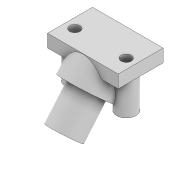
# Autodesk Inventor part: Landing_leg_clamp_large
Saved by Autodesk Inventor 2022 (Build 260153000, 153)
## iProperties
Created: 2022-05-01
Part Number: Landing_leg_clamp_large
Material: Generic
Document SubType Name: Modeling
Designer: dell
Density: 1 g/cm^3
Appearance: Default
Mass: 2.35409 g
Surface Area: 17.5445 cm^2
Volume: 2.35409 cm^3
Author: dell
Autodesk Inventor part; units mm, degrees
ref_plane "YZ Plane" through (0, 0, 0) normal (1, 0, 0) x (0, 1, 0)
ref_plane "XZ Plane" through (0, 0, 0) normal (0, 1, 0) x (-1, 0, 0)
ref_plane "XY Plane" through (0, 0, 0) normal (0, 0, 1) x (1, 0, 0)
sketch "Sketch6" plane through (0, 0, 0) normal (0, 1, 0) x (-1, 0, 0)
  line L0 (0, 0) -> (22, 0)
  line L1 (22, 0) -> (22, -14)
  line L2 (22, -14) -> (0, -14)
  line L3 (0, -14) -> (0, 0)
  dimension "d29" = 22
  dimension "d30" = 14
  constraints: 8 end point, 2 parallel, 1 horizontal, 1 perpendicular
  measures "d29" distance of L0.start L0.end
  measures "d30" distance between parallel lines of L0 L2
extrude "Extrusion6" add sketch "Sketch6" along normal blind 4
ref_plane "Work Plane3" through (-22, 0, 0) normal (0, -0.7660444, 0.6427876) x (1, 0, 0)
sketch "Sketch7" plane through (-22, 0, 0) normal (0, -0.7660444, 0.6427876) x (1, 0, 0)
  circle A0 centre (11, -5) radius 1.5
  line L0 (0, 0) -> (0, 2.5712) projected
  circle A1 centre (11, -5) radius 4.9
  point P0 (22, 0)
  dimension "d34" = 3
  dimension "d35" = 5
  dimension "d36" = 11
  dimension "d37" = 9.8
  constraints: 2 centre point, 1 coincident
  measures "d34" diameter of A0
  measures "d35" vertical distance of point (22, 0) A0.centre
  measures "d36" distance from line of L0 A0.centre
  measures "d37" diameter of A1
extrude "Extrusion7" add sketch "Sketch7" along normal blind 15 and the other way blind 20
sketch "Sketch9" plane through (0, 0, 0) normal (0, -1, 0) x (1, 0, 0)
  circle A0 centre (-19, -5.5) radius 1.6
  circle A1 centre (-3, -5.5) radius 1.6
  line L0 (-22, 0) -> (0, 0) projected
  line L1 (-22, 0) -> (0, 0) projected
  line L2 (-22, -14) -> (-22, 0) projected
  line L3 (0, 0) -> (0, -14) projected
  dimension "d43" = 3.2
  dimension "d44" = 3.2
  dimension "d45" = 5.5
  dimension "d46" = 5.5
  dimension "d47" = 3
  dimension "d48" = 3
  constraints: 2 centre point
  measures "d43" diameter of A0
  measures "d44" diameter of A1
  measures "d45" distance from line of L0 A0.centre
  measures "d46" distance from line of L1 A1.centre
  measures "d47" distance from line of L2 A0.centre
  measures "d48" distance from line of L3 A1.centre
extrude "Extrusion9" cut sketch "Sketch9" along normal mid plane 10
ref_plane "Work Plane4" through (-11, -3.2139, -3.8302) normal (0, -0.7660444, 0.6427876) x (-1, 0, 0)
sketch "Sketch20" plane through (-11, -3.2139, -3.8302) normal (0, -0.7660444, 0.6427876) x (-1, 0, 0)
  circle A0 centre (0, 0) radius 4.9 projected
  circle A1 centre (0, 0) radius 1.5 projected
  circle A2 centre (0, 0) radius 6.1
  circle A3 centre (0, 0) radius 7.5
  point P0 (-11, -5)
  dimension "d87" = 12.2
  dimension "d88" = 15
  constraints: 2 centre point, 2 coincident
  measures "d87" diameter of A2
  measures "d88" diameter of A3
sketch "Sketch26" plane through (0, 0, 0) normal (0, -1, 0) x (1, 0, 0)
  circle A0 centre (-3, -5.5) radius 1.6 projected
  circle A1 centre (-19, -5.5) radius 1.6 projected
  line L0 (0, -14) -> (-22, -14) projected
  line L1 (0, 0) -> (0, -14) projected
  line L2 (-22, 0) -> (0, 0) projected
  line L3 (-22, -14) -> (-22, 0) projected
  ellipse E0 centre (-11, -6.527) end of major axis (-11, -0.1305) minor radius 4.9 projected
  circle A2 centre (-19, -5.5) radius 3
  circle A3 centre (-3, -5.5) radius 3
  dimension "d105" = 6
  dimension "d106" = 6
  constraints: 2 centre point, 2 coincident, 1 other
  measures "d105" diameter of A2
  measures "d106" diameter of A3
extrude "Extrusion25" add sketch "Sketch26" along normal blind 10 contours A3 | A2
extrude "Extrusion19" cut sketch "Sketch20" along normal mid plane 8 contours A2
extrude "Extrusion20" add sketch "Sketch20" along normal blind 4 and the other way blind 20 contours A3
sketch "Sketch22" plane through (0, 4, 0) normal (0, 1, 0) x (1, 0, 0)
  arc A0 (-18.129, 6.8421) -> (-17.4889, 4.974) centre (-19, 5.5) ccw projected
  arc A1 (-4.5111, 4.974) -> (-3.871, 6.8421) centre (-3, 5.5) ccw projected
  circle A2 centre (-3, 5.5) radius 1.6
  circle A3 centre (-19, 5.5) radius 1.6
  point P0 (0, 0)
  point P1 (-3.871, 6.8421)
  point P2 (-4.5111, 4.974)
  point P3 (-18.129, 6.8421)
  constraints: 2 centre point, 2 coincident, 2 concentric
extrude "Extrusion22" cut sketch "Sketch22" against normal blind 100
sketch "Sketch23" plane through (-11, -0.1498, -6.4014) normal (0, -0.7660444, 0.6427876) x (1, 0, 0)
  circle A0 centre (0, 0) radius 6.1 projected
  circle A1 centre (0, 0) radius 4.9 projected
  point P0 (11, 5)
extrude "Extrusion23" add sketch "Sketch23" against normal blind 100
sketch "Sketch27" plane through (0, 0, -14) normal (1, 0, 0) x (0, 0, -1)
  line L0 (-14, 0) -> (-14, 4) projected
  line L1 (0, 4) -> (0, 0) projected
  line L2 (-14, 4) -> (0, 4)
  line L3 (0, 4) -> (0, -6.5028)
  line L4 (0, -6.5028) -> (99.7607, -6.5028)
  line L5 (99.7607, -6.5028) -> (99.7607, 91.2671)
  line L6 (99.7607, 91.2671) -> (-14, 91.2671)
  line L7 (-14, 91.2671) -> (-14, 4)
  constraints: 12 end point, 5 perpendicular, 1 horizontal
extrude "Extrusion26" cut sketch "Sketch27" against normal blind 100
sketch "Sketch28" plane through (0, -10, 0) normal (0, -1, 0) x (1, 0, 0)
  circle A0 centre (-19, -5.5) radius 3 projected
  circle A1 centre (-19, -5.5) radius 1.6 projected
  circle A2 centre (-3, -5.5) radius 3 projected
  circle A3 centre (-3, -5.5) radius 1.6 projected
  point P0 (0, 0)
body "Solid2"
